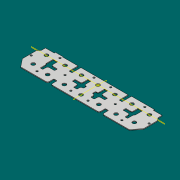
# Autodesk Inventor part: pcb_middle
Saved by Autodesk Inventor 2018 (Build 220112000, 112)
## iProperties
Created: 2021-10-17
Part Number: pcb_middle
Material: アルミニウム 6061
Document SubType Name: Modeling
Designer: gisen
Density: 2.7 g/cm^3
Appearance: アルミニウム - フラット
Author: gisen
Autodesk Inventor part; units mm, degrees
ref_plane "XY Plane" through (0, 0, 0) normal (0, 0, 1) x (1, 0, 0)
sketch "スケッチ1" plane through (0, 0, 0) normal (0, 0, 1) x (1, 0, 0)
  arc A0 (-25.2, 7.4139) -> (-26.2, 6.4139) centre (-25.2, 6.4139) ccw construction
  arc A1 (-19, 3.9139) -> (-21, 3.9139) centre (-20, 3.9139) ccw construction
  arc A2 (-10.8, 6.4139) -> (-11.8, 7.4139) centre (-11.8, 6.4139) ccw construction
  arc A3 (-6.7, 7.4139) -> (-7.7, 6.4139) centre (-6.7, 6.4139) ccw construction
  arc A4 (7.7, 6.4139) -> (6.7, 7.4139) centre (6.7, 6.4139) ccw construction
  arc A5 (11.8, 7.4139) -> (10.8, 6.4139) centre (11.8, 6.4139) ccw construction
  arc A6 (26.2, 6.4139) -> (25.2, 7.4139) centre (25.2, 6.4139) ccw construction
  line L0 (-67.1, -22.0601) -> (-67.1, -6.6726)
  line L1 (-67.1, -6.6726) -> (-64.6, -3.5297)
  line L2 (-64.6, -3.5297) -> (-64.6, 0.9639)
  line L3 (-64.6, 2.3139) -> (-54.9, 2.3139) construction
  line L4 (-29.4, 2.3139) -> (-29.4, 1.8139) construction
  line L5 (-28.8, -8.1959) -> (-26.7, -8.1959)
  line L6 (-26.1, -7.5959) -> (-26.1, 1.8139)
  line L7 (-26.1, 2.3139) -> (26.1, 2.3139) construction
  line L8 (26.1, 2.3139) -> (26.1, 1.8139)
  line L9 (26.7, -8.1959) -> (28.8, -8.1959)
  line L10 (29.4, -7.5959) -> (29.4, 2.3139)
  line L11 (29.4, 2.3139) -> (54.8, 2.3139)
  line L12 (64.6, 2.3139) -> (64.6, 0.9639) construction
  line L13 (64.6, -3.5297) -> (67.1, -6.6726)
  line L14 (67.1, -6.6726) -> (67.1, -22.0601)
  line L15 (67.1, -22.0601) -> (60.0795, -30.8861)
  line L16 (60.0795, -30.8861) -> (32, -30.8861)
  line L17 (30.3, -29.1861) -> (30.3, -24.5959)
  line L18 (29.7, -23.9959) -> (27.3, -23.9959)
  line L19 (26.7, -24.5959) -> (26.7, -29.1861)
  line L20 (25, -30.8861) -> (-25, -30.8861)
  line L21 (-26.7, -29.1861) -> (-26.7, -24.5959)
  line L22 (-27.3, -23.9959) -> (-29.7, -23.9959)
  line L23 (-30.3, -24.5959) -> (-30.3, -29.1861)
  line L24 (-32, -30.8861) -> (-60.0795, -30.8861)
  line L25 (-60.0795, -30.8861) -> (-67.1, -22.0601)
  line L26 (-64.5913, -25.214) -> (-66.9913, -22.1968) construction
  line L27 (64.5913, -25.214) -> (66.9913, -22.1968) construction
  line L28 (-66.0851, -5.2361) -> (-64.8087, -3.6314) construction
  line L29 (-67.1, -21.8855) -> (-67.1, -5.0802) construction
  line L30 (67.1, -5.0802) -> (67.1, -21.8855) construction
  line L31 (64.8087, -3.6314) -> (66.0851, -5.2361) construction
  line L32 (-45.0166, 2.4139) -> (-54.9, 2.4139) construction
  line L33 (54.8, 2.4139) -> (45.0166, 2.4139) construction
  arc A7 (-26.2, 0.8639) -> (-29.3, 0.8639) centre (-27.75, 0.8639) ccw construction
  line L34 (-45.0166, 2.4139) -> (-27.75, 2.4139) construction
  line L35 (-27.75, 2.4139) -> (-27.75, 0.8639) construction
  line L36 (-64.7, -3.3202) -> (-64.7, 0.0639) construction
  line L37 (64.7, 0.0639) -> (64.7, -3.3202) construction
  arc A8 (-32, -30.8861) -> (-30.3, -29.1861) centre (-32, -29.1861) ccw
  arc A9 (-26.7, -29.1861) -> (-25, -30.8861) centre (-25, -29.1861) ccw
  arc A10 (25, -30.8861) -> (26.7, -29.1861) centre (25, -29.1861) ccw
  arc A11 (30.3, -29.1861) -> (32, -30.8861) centre (32, -29.1861) ccw
  arc A12 (-32, -30.9861) -> (-30.2, -29.1861) centre (-32, -29.1861) ccw construction
  arc A13 (25, -31.2861) -> (26.8, -29.4861) centre (25, -29.4861) ccw construction
  arc A14 (30.2, -29.1861) -> (32, -30.9861) centre (32, -29.1861) ccw construction
  arc A15 (-26.8, -29.4861) -> (-25, -31.2861) centre (-25, -29.4861) ccw construction
  arc A16 (-29.7, -24.0959) -> (-30.2, -24.5959) centre (-29.7, -24.5959) ccw construction
  arc A17 (-26.8, -24.5959) -> (-27.3, -24.0959) centre (-27.3, -24.5959) ccw construction
  arc A18 (27.3, -24.0959) -> (26.8, -24.5959) centre (27.3, -24.5959) ccw construction
  arc A19 (30.2, -24.5959) -> (29.7, -24.0959) centre (29.7, -24.5959) ccw construction
  line L38 (-26.7, -8.0959) -> (-28.8, -8.0959) construction
  arc A20 (-29.4, -7.5959) -> (-28.8, -8.1959) centre (-28.8, -7.5959) ccw
  arc A21 (-26.7, -8.1959) -> (-26.1, -7.5959) centre (-26.7, -7.5959) ccw
  arc A22 (-29.3, -7.5959) -> (-28.8, -8.0959) centre (-28.8, -7.5959) ccw construction
  arc A23 (-26.7, -8.0959) -> (-26.2, -7.5959) centre (-26.7, -7.5959) ccw construction
  arc A24 (-29.7, -23.9959) -> (-30.3, -24.5959) centre (-29.7, -24.5959) ccw
  arc A25 (-26.7, -24.5959) -> (-27.3, -23.9959) centre (-27.3, -24.5959) ccw
  arc A26 (27.3, -23.9959) -> (26.7, -24.5959) centre (27.3, -24.5959) ccw
  arc A27 (30.3, -24.5959) -> (29.7, -23.9959) centre (29.7, -24.5959) ccw
  arc A28 (29.3, 0.8639) -> (26.2, 0.8639) centre (27.75, 0.8639) ccw construction
  arc A29 (26.2, -7.5959) -> (26.7, -8.0959) centre (26.7, -7.5959) ccw construction
  arc A30 (28.8, -8.0959) -> (29.3, -7.5959) centre (28.8, -7.5959) ccw construction
  arc A31 (26.1, -7.5959) -> (26.7, -8.1959) centre (26.7, -7.5959) ccw
  arc A32 (28.8, -8.1959) -> (29.4, -7.5959) centre (28.8, -7.5959) ccw
  line L39 (-26.1, 1.8139) -> (26.1, 1.8139)
  line L40 (-26.1, 1.8139) -> (-26.1, 2.3139) construction
  line L41 (26.1, 1.8139) -> (26.1, -7.5959)
  circle A33 centre (-47, -0.5861) radius 0.8 construction
  circle A34 centre (-65.2959, -14.0786) radius 0.8 construction
  circle A35 centre (-46.95, -25.9861) radius 0.8 construction
  circle A36 centre (-27.8915, -14.0959) radius 0.8 construction
  circle A37 centre (-9.25, -0.5861) radius 0.8 construction
  circle A38 centre (9.25, -0.5861) radius 0.8 construction
  circle A39 centre (27.8915, -14.0959) radius 0.8 construction
  circle A40 centre (9.55, -25.9861) radius 0.8 construction
  circle A41 centre (-9.55, -25.9861) radius 0.8 construction
  circle A42 centre (46.95, -25.9861) radius 0.8 construction
  circle A43 centre (47, -0.5861) radius 0.8 construction
  circle A44 centre (65.2959, -14.0786) radius 0.8 construction
  line L42 (-48.8, -5.4861) -> (-45.2, -5.4861)
  line L43 (-44.6, -6.0861) -> (-44.6, -10.7861)
  line L44 (-42.9, -12.4861) -> (-38.3915, -12.4861)
  line L45 (-37.7915, -13.0861) -> (-37.7915, -15.0861)
  line L46 (-38.3915, -15.6861) -> (-43.8, -15.6861)
  line L47 (-45.5, -17.3861) -> (-45.5, -20.4861)
  line L48 (-46.1, -21.0861) -> (-47.8, -21.0861)
  line L49 (-48.4, -20.4861) -> (-48.4, -15.2861)
  arc A45 (-48.4, -15.2861) -> (-49.1391, -13.8837) centre (-50.1, -15.2861) ccw
  arc A46 (-48.3, -15.2861) -> (-48.5711, -14.3361) centre (-50.1, -15.2861) ccw construction
  arc A47 (-49.4, -13.3887) -> (-49.1391, -13.8837) centre (-48.8, -13.3887) ccw
  line L50 (-49.4, -6.0861) -> (-49.4, -13.3887)
  arc A48 (-49.3, -13.3887) -> (-49.0826, -13.8012) centre (-48.8, -13.3887) ccw construction
  arc A49 (-48.8, -5.5861) -> (-49.3, -6.0861) centre (-48.8, -6.0861) ccw construction
  arc A50 (-44.7, -6.0861) -> (-45.2, -5.5861) centre (-45.2, -6.0861) ccw construction
  arc A51 (-44.7, -10.7861) -> (-44.5015, -11.6078) centre (-42.9, -10.7861) ccw construction
  arc A52 (-37.8915, -13.0861) -> (-38.3915, -12.5861) centre (-38.3915, -13.0861) ccw construction
  arc A53 (-38.3915, -15.5861) -> (-37.8915, -15.0861) centre (-38.3915, -15.0861) ccw construction
  arc A54 (-43.8, -15.5861) -> (-45.6, -17.3861) centre (-43.8, -17.3861) ccw construction
  arc A55 (-46.1, -20.9861) -> (-45.6, -20.4861) centre (-46.1, -20.4861) ccw construction
  arc A56 (-48.3, -20.4861) -> (-47.8, -20.9861) centre (-47.8, -20.4861) ccw construction
  arc A57 (-48.8, -5.4861) -> (-49.4, -6.0861) centre (-48.8, -6.0861) ccw
  arc A58 (-44.6, -6.0861) -> (-45.2, -5.4861) centre (-45.2, -6.0861) ccw
  arc A59 (-48.4, -20.4861) -> (-47.8, -21.0861) centre (-47.8, -20.4861) ccw
  arc A60 (-46.1, -21.0861) -> (-45.5, -20.4861) centre (-46.1, -20.4861) ccw
  arc A61 (-38.3915, -15.6861) -> (-37.7915, -15.0861) centre (-38.3915, -15.0861) ccw
  arc A62 (-37.7915, -13.0861) -> (-38.3915, -12.4861) centre (-38.3915, -13.0861) ccw
  arc A63 (-44.6, -10.7861) -> (-42.9, -12.4861) centre (-42.9, -10.7861) ccw
  arc A64 (-43.8, -15.6861) -> (-45.5, -17.3861) centre (-43.8, -17.3861) ccw
  arc A65 (-17.3915, -12.8861) -> (-17.8915, -13.3861) centre (-17.3915, -13.3861) ccw construction
  arc A66 (-17.8915, -15.3861) -> (-17.3915, -15.8861) centre (-17.3915, -15.3861) ccw construction
  arc A67 (-12.6, -12.8861) -> (-10.8984, -11.673) centre (-12.6, -11.0861) ccw construction
  arc A68 (-11.4, -17.6861) -> (-13.2, -15.8861) centre (-13.2, -17.6861) ccw construction
  arc A69 (-5.9, -16.4861) -> (-7.7, -18.2861) centre (-5.9, -18.2861) ccw construction
  arc A70 (-7.6652, -11.7382) -> (-5.9, -13.1861) centre (-5.9, -11.3861) ccw construction
  arc A71 (-10.3, -5.5861) -> (-10.8, -6.0861) centre (-10.3, -6.0861) ccw construction
  arc A72 (-7.7, -6.0861) -> (-8.2, -5.5861) centre (-8.2, -6.0861) ccw construction
  arc A73 (-5.5, -16.4861) -> (-5, -15.9861) centre (-5.5, -15.9861) ccw construction
  arc A74 (-5, -13.6861) -> (-5.5, -13.1861) centre (-5.5, -13.6861) ccw construction
  arc A75 (-8.2, -20.9861) -> (-7.7, -20.4861) centre (-8.2, -20.4861) ccw construction
  arc A76 (-11.4, -20.4861) -> (-10.9, -20.9861) centre (-10.9, -20.4861) ccw construction
  line L51 (-10.9, -11.0861) -> (-10.9, -6.0861)
  line L52 (-10.3, -5.4861) -> (-8.2, -5.4861)
  line L53 (-7.6, -6.0861) -> (-7.6, -11.3861)
  line L54 (-5.9, -13.0861) -> (-5.5, -13.0861)
  line L55 (-4.9, -13.6861) -> (-4.9, -15.9861)
  line L56 (-5.5, -16.5861) -> (-5.9, -16.5861)
  line L57 (-7.6, -18.2861) -> (-7.6, -20.4861)
  line L58 (-8.2, -21.0861) -> (-10.9, -21.0861)
  line L59 (-11.5, -20.4861) -> (-11.5, -17.6861)
  line L60 (-13.2, -15.9861) -> (-17.3915, -15.9861)
  line L61 (-17.9915, -15.3861) -> (-17.9915, -13.3861)
  line L62 (-17.3915, -12.7861) -> (-12.6, -12.7861)
  arc A77 (-11.5, -20.4861) -> (-10.9, -21.0861) centre (-10.9, -20.4861) ccw
  arc A78 (-8.2, -21.0861) -> (-7.6, -20.4861) centre (-8.2, -20.4861) ccw
  arc A79 (-5.5, -16.5861) -> (-4.9, -15.9861) centre (-5.5, -15.9861) ccw
  arc A80 (-4.9, -13.6861) -> (-5.5, -13.0861) centre (-5.5, -13.6861) ccw
  arc A81 (-7.6, -6.0861) -> (-8.2, -5.4861) centre (-8.2, -6.0861) ccw
  arc A82 (-10.3, -5.4861) -> (-10.9, -6.0861) centre (-10.3, -6.0861) ccw
  arc A83 (-17.3915, -12.7861) -> (-17.9915, -13.3861) centre (-17.3915, -13.3861) ccw
  arc A84 (-17.9915, -15.3861) -> (-17.3915, -15.9861) centre (-17.3915, -15.3861) ccw
  arc A85 (-12.6, -12.7861) -> (-10.9, -11.0861) centre (-12.6, -11.0861) ccw
  arc A86 (-7.6, -11.3861) -> (-5.9, -13.0861) centre (-5.9, -11.3861) ccw
  arc A87 (-5.9, -16.5861) -> (-7.6, -18.2861) centre (-5.9, -18.2861) ccw
  arc A88 (-11.5, -17.6861) -> (-13.2, -15.9861) centre (-13.2, -17.6861) ccw
  line L63 (0, 1.8139) -> (0, -30.8861) construction
  line L64 (48.8, -5.4861) -> (45.2, -5.4861)
  line L65 (44.6, -6.0861) -> (44.6, -10.7861)
  line L66 (42.9, -12.4861) -> (38.3915, -12.4861)
  line L67 (37.7915, -13.0861) -> (37.7915, -15.0861)
  line L68 (38.3915, -15.6861) -> (43.8, -15.6861)
  line L69 (45.5, -17.3861) -> (45.5, -20.4861)
  line L70 (46.1, -21.0861) -> (47.8, -21.0861)
  line L71 (48.4, -20.4861) -> (48.4, -15.2861)
  arc A89 (49.1391, -13.8837) -> (48.4, -15.2861) centre (50.1, -15.2861) ccw
  arc A90 (49.1391, -13.8837) -> (49.4, -13.3887) centre (48.8, -13.3887) ccw
  line L72 (49.4, -6.0861) -> (49.4, -13.3887)
  arc A91 (49.4, -6.0861) -> (48.8, -5.4861) centre (48.8, -6.0861) ccw
  arc A92 (45.2, -5.4861) -> (44.6, -6.0861) centre (45.2, -6.0861) ccw
  arc A93 (47.8, -21.0861) -> (48.4, -20.4861) centre (47.8, -20.4861) ccw
  arc A94 (45.5, -20.4861) -> (46.1, -21.0861) centre (46.1, -20.4861) ccw
  arc A95 (37.7915, -15.0861) -> (38.3915, -15.6861) centre (38.3915, -15.0861) ccw
  arc A96 (38.3915, -12.4861) -> (37.7915, -13.0861) centre (38.3915, -13.0861) ccw
  arc A97 (42.9, -12.4861) -> (44.6, -10.7861) centre (42.9, -10.7861) ccw
  arc A98 (45.5, -17.3861) -> (43.8, -15.6861) centre (43.8, -17.3861) ccw
  line L73 (10.9, -11.0861) -> (10.9, -6.0861)
  line L74 (10.3, -5.4861) -> (8.2, -5.4861)
  line L75 (7.6, -6.0861) -> (7.6, -11.3861)
  line L76 (5.9, -13.0861) -> (5.5, -13.0861)
  line L77 (4.9, -13.6861) -> (4.9, -15.9861)
  line L78 (7.6, -18.2861) -> (7.6, -20.4861)
  line L79 (8.2, -21.0861) -> (10.9, -21.0861)
  line L80 (11.5, -20.4861) -> (11.5, -17.6861)
  line L81 (13.2, -15.9861) -> (17.3915, -15.9861)
  line L82 (17.9915, -15.3861) -> (17.9915, -13.3861)
  line L83 (17.3915, -12.7861) -> (12.6, -12.7861)
  arc A99 (10.9, -21.0861) -> (11.5, -20.4861) centre (10.9, -20.4861) ccw
  arc A100 (7.6, -20.4861) -> (8.2, -21.0861) centre (8.2, -20.4861) ccw
  arc A101 (4.9, -15.9861) -> (5.5, -16.5861) centre (5.5, -15.9861) ccw
  arc A102 (5.5, -13.0861) -> (4.9, -13.6861) centre (5.5, -13.6861) ccw
  arc A103 (8.2, -5.4861) -> (7.6, -6.0861) centre (8.2, -6.0861) ccw
  arc A104 (10.9, -6.0861) -> (10.3, -5.4861) centre (10.3, -6.0861) ccw
  arc A105 (17.9915, -13.3861) -> (17.3915, -12.7861) centre (17.3915, -13.3861) ccw
  arc A106 (17.3915, -15.9861) -> (17.9915, -15.3861) centre (17.3915, -15.3861) ccw
  arc A107 (10.9, -11.0861) -> (12.6, -12.7861) centre (12.6, -11.0861) ccw
  arc A108 (5.9, -13.0861) -> (7.6, -11.3861) centre (5.9, -11.3861) ccw
  arc A109 (7.6, -18.2861) -> (5.9, -16.5861) centre (5.9, -18.2861) ccw
  arc A110 (13.2, -15.9861) -> (11.5, -17.6861) centre (13.2, -17.6861) ccw
  circle A111 centre (-65.2959, -14.0786) radius 1.05
  circle A112 centre (-47, -0.5861) radius 1.05
  circle A113 centre (-46.95, -25.9861) radius 1.05
  circle A114 centre (-27.8915, -14.0959) radius 1.05
  circle A115 centre (-9.25, -0.5861) radius 1.05
  circle A116 centre (-9.55, -25.9861) radius 1.05
  circle A117 centre (9.55, -25.9861) radius 1.05
  circle A118 centre (9.25, -0.5861) radius 1.05
  circle A119 centre (27.8915, -14.0959) radius 1.05
  circle A120 centre (46.95, -25.9861) radius 1.05
  circle A121 centre (47, -0.5861) radius 1.05
  circle A122 centre (65.2959, -14.0786) radius 1.05
  line L84 (5.5, -16.5861) -> (5.9, -16.5861)
  line L85 (-64.6, 0.9639) -> (-54.9, 0.9639)
  line L86 (-54.9, 0.9639) -> (-54.9, 2.3139)
  line L87 (-55, 14.0639) -> (-55, 2.7139) construction
  line L88 (-65.7, 1.0639) -> (-66.1, 1.0639) construction
  line L89 (-54.9, 2.3139) -> (-46.4, 2.3139)
  line L90 (-64.6, 0.9639) -> (-64.6, 2.3139) construction
  line L91 (54.9, 2.7139) -> (54.9, 11.2639) construction
  line L92 (66.1, 1.0639) -> (65.7, 1.0639) construction
  line L93 (54.8, 2.3139) -> (54.8, 0.9639)
  line L94 (54.8, 0.9639) -> (64.6, 0.9639)
  line L95 (54.8, 2.3139) -> (64.6, 2.3139) construction
  line L96 (64.6, 0.9639) -> (64.6, -3.5297)
  line L97 (-46.4, 2.3139) -> (-46.4, 1.8139)
  line L98 (-46.4, 1.8139) -> (-29.4, 1.8139)
  line L99 (-46.3, 14.0639) -> (-46.3, 3.1139) construction
  line L100 (-29.4, 1.8139) -> (-29.4, -7.5959)
  line L101 (-46.4, 2.3139) -> (-29.4, 2.3139) construction
  point P0 (0, 0)
  point P1 (26.7, -30.8861)
  point P2 (-26.7, -30.8861)
  point P3 (-30.3, -30.8861)
  dimension "d1" = 0.1
  dimension "d3" = 0.1
  dimension "d4" = 0.1
  dimension "d6" = 0.1
  dimension "d7" = 0.1
  dimension "d8" = 0.1
  dimension "d9" = 0.1
  dimension "d10" = 0.1
  dimension "d11" = 0.1
  dimension "d12" = 0.1
  dimension "d13" = 0.1
  dimension "d18" = 0.1
  dimension "d19" = 0.1
  dimension "d21" = 0.5
  dimension "d22" = 0.1
  dimension "d25" = 0.1
  dimension "d28" = 2.1
  dimension "d31" = 0.1
  dimension "d32" = 0.1
  dimension "d33" = 0.5
  dimension "d34" = 0.1
  dimension "d35" = 0.1
  dimension "d36" = 0.1
  constraints: 172 end point, 112 point on circle, 70 tangent, 68 centre point, 65 symmetric about line, 59 perpendicular, 34 equal radius, 33 coincident, 15 point on line, 9 vertical, 5 parallel, 4 horizontal, 2 collinear, 2 midpoint, 22 other
  measures "d1" distance from line of A16.end L23
  measures "d3" distance from line of L21 A17.start
  measures "d4" distance from line of L19 A18.end
  measures "d6" distance from line of A19.start L17
  measures "d7" distance from line of L28.start L1
  measures "d8" distance from line of L1.end L36
  measures "d9" distance from line of L3 L32.start
  measures "d10" distance from line of L37.start L12
  measures "d11" distance between parallel lines of L31 L13
  measures "d12" distance from line of A7.end L4
  measures "d13" distance from line of A7.start L6
  measures "d18" distance from line of A29.start L8
  measures "d19" distance from line of A30.end L10
  measures "d21" distance from line of L7 L6.end
  measures "d22" distance from line of L50 A49.end
  measures "d25" distance from line of L59 A76.start
  measures "d28" diameter of A111
  measures "d31" distance between parallel lines of L88 L85
  measures "d32" distance between parallel lines of L92 L94
  measures "d33" distance between parallel lines of L89 L98
  measures "d34" distance between parallel lines of L86 L87
  measures "d35" distance between parallel lines of L97 L99
  measures "d36" distance between parallel lines of L91 L93
extrude "押し出し1" add sketch "スケッチ1" along normal blind 0.8
sketch "スケッチ2" plane through (0, 0, 0.8) normal (0, 0, 1) x (1, 0, 0)
  arc A0 (-49.3, 0.4139) -> (-51.1, 2.2139) centre (-51.1, 0.4139) ccw construction
  arc A1 (-64.7, -11.3861) -> (-63.1942, -13.1618) centre (-62.9, -11.3861) ccw construction
  arc A2 (-63.0124, -13.8709) -> (-63.7, -15.2861) centre (-61.9, -15.2861) ccw construction
  arc A3 (-50.1, -28.8861) -> (-48.3, -27.0861) centre (-50.1, -27.0861) ccw construction
  arc A4 (-43.8, -15.5861) -> (-45.6, -17.3861) centre (-43.8, -17.3861) ccw construction
  arc A5 (-32, -30.9861) -> (-30.2, -29.1861) centre (-32, -29.1861) ccw construction
  arc A6 (-25, -15.8861) -> (-26.8, -17.6861) centre (-25, -17.6861) ccw construction
  arc A7 (-13.2, -31.2861) -> (-11.4, -29.4861) centre (-13.2, -29.4861) ccw construction
  arc A8 (-5.9, -16.4861) -> (-7.7, -18.2861) centre (-5.9, -18.2861) ccw construction
  arc A9 (6.6435, -31.7253) -> (7.7, -30.0861) centre (5.9, -30.0861) ccw construction
  arc A10 (-29.3, 1.0139) -> (-29.3522, 1.4444) centre (-31.1, 1.0139) ccw construction
  arc A11 (-44.5015, -11.6078) -> (-42.9, -12.5861) centre (-42.9, -10.7861) ccw construction
  arc A12 (-26.1016, -11.673) -> (-24.4, -12.8861) centre (-24.4, -11.0861) ccw construction
  arc A13 (-10.9274, 1.3792) -> (-12.6, 2.5139) centre (-12.6, 0.7139) ccw construction
  arc A14 (-7.4588, 1.3139) -> (-7.7, 0.4139) centre (-5.9, 0.4139) ccw construction
  arc A15 (5.9, -13.1861) -> (7.6652, -11.7382) centre (5.9, -11.3861) ccw construction
  arc A16 (10.9274, 1.3792) -> (10.8, 0.7139) centre (12.6, 0.7139) ccw construction
  arc A17 (26.1016, -11.673) -> (26.2, -11.0861) centre (24.4, -11.0861) ccw construction
  arc A18 (31.1, 2.8139) -> (29.3522, 1.4444) centre (31.1, 1.0139) ccw construction
  arc A19 (44.5015, -11.6078) -> (44.7, -10.7861) centre (42.9, -10.7861) ccw construction
  arc A20 (51.1, 2.2139) -> (49.3, 0.4139) centre (51.1, 0.4139) ccw construction
  arc A21 (63.1942, -13.1618) -> (64.7, -11.3861) centre (62.9, -11.3861) ccw construction
  arc A22 (48.3, -27.0861) -> (49.825, -28.8649) centre (50.1, -27.0861) ccw construction
  arc A23 (63.7, -15.2861) -> (63.0124, -13.8709) centre (61.9, -15.2861) ccw construction
  arc A24 (45.6, -17.3861) -> (43.8, -15.5861) centre (43.8, -17.3861) ccw construction
  arc A25 (15.8, -58.8861) -> (15.2, -58.2861) centre (15.2, -58.8861) ccw construction
  line L0 (15.8, -58.8861) -> (15.8, -62.2861) construction
  arc A26 (15.2, -62.8861) -> (15.8, -62.2861) centre (15.2, -62.2861) ccw construction
  line L1 (15.2, -62.8861) -> (8.2, -62.8861) construction
  arc A27 (7.6, -62.2861) -> (8.2, -62.8861) centre (8.2, -62.2861) ccw construction
  line L2 (7.6, -62.2861) -> (7.6, -58.8861) construction
  arc A28 (8.2, -58.2861) -> (7.6, -58.8861) centre (8.2, -58.8861) ccw construction
  line L3 (8.2, -58.2861) -> (15.2, -58.2861) construction
  arc A29 (-7.6, -58.8861) -> (-8.2, -58.2861) centre (-8.2, -58.8861) ccw construction
  line L4 (-7.6, -58.8861) -> (-7.6, -62.2861) construction
  arc A30 (-8.2, -62.8861) -> (-7.6, -62.2861) centre (-8.2, -62.2861) ccw construction
  line L5 (-8.2, -62.8861) -> (-15.2, -62.8861) construction
  arc A31 (-15.8, -62.2861) -> (-15.2, -62.8861) centre (-15.2, -62.2861) ccw construction
  line L6 (-15.8, -62.2861) -> (-15.8, -58.8861) construction
  arc A32 (-15.2, -58.2861) -> (-15.8, -58.8861) centre (-15.2, -58.8861) ccw construction
  line L7 (-15.2, -58.2861) -> (-8.2, -58.2861) construction
  arc A33 (-3.85, -54.4861) -> (-3.25, -55.0861) centre (-3.25, -54.4861) ccw construction
  line L8 (-3.85, -54.4861) -> (-3.85, -53.2461) construction
  arc A34 (-3.25, -52.6461) -> (-3.85, -53.2461) centre (-3.25, -53.2461) ccw construction
  line L9 (-3.25, -52.6461) -> (3.25, -52.6461) construction
  arc A35 (3.85, -53.2461) -> (3.25, -52.6461) centre (3.25, -53.2461) ccw construction
  line L10 (3.85, -53.2461) -> (3.85, -54.4861) construction
  arc A36 (3.25, -55.0861) -> (3.85, -54.4861) centre (3.25, -54.4861) ccw construction
  line L11 (3.25, -55.0861) -> (-3.25, -55.0861) construction
  circle A37 centre (30.05, -39.9861) radius 1.05 construction
  circle A38 centre (38.492, -53.6861) radius 1.05 construction
  circle A39 centre (11.7, -65.7861) radius 1.05 construction
  circle A40 centre (9.75, -53.1361) radius 1.05 construction
  circle A41 centre (-9.75, -53.1361) radius 1.05 construction
  circle A42 centre (-11.7, -65.7861) radius 1.05 construction
  circle A43 centre (-38.492, -53.6861) radius 1.05 construction
  circle A44 centre (-30.05, -39.9861) radius 1.05 construction
  line L12 (-27.3621, -37.0861) -> (-32.4, -37.0861) construction
  arc A45 (-33, -36.4861) -> (-32.4, -37.0861) centre (-32.4, -36.4861) ccw construction
  line L13 (-33, -36.4861) -> (-33, -31.3861) construction
  arc A46 (-33, -31.3861) -> (-33.9, -30.4861) centre (-33.9, -31.3861) ccw construction
  line L14 (-33.9, -30.4861) -> (-44.6, -30.4861) construction
  arc A47 (-44.6, -30.4861) -> (-45.5, -31.3861) centre (-44.6, -31.3861) ccw construction
  line L15 (-45.5, -31.3861) -> (-45.5, -34.7861) construction
  arc A48 (-46.1, -35.3861) -> (-45.5, -34.7861) centre (-46.1, -34.7861) ccw construction
  line L16 (-46.1, -35.3861) -> (-46.5, -35.3861) construction
  arc A49 (-46.5, -35.3861) -> (-48.2, -37.0861) centre (-46.5, -37.0861) ccw construction
  line L17 (-48.2, -37.0861) -> (-48.2, -48.8861) construction
  arc A50 (-48.2, -48.8861) -> (-46.5, -50.5861) centre (-46.5, -48.8861) ccw construction
  line L18 (-46.5, -50.5861) -> (-46.1031, -50.5861) construction
  arc A51 (-45.6678, -50.773) -> (-46.1031, -50.5861) centre (-46.1031, -51.1861) ccw construction
  line L19 (-45.6678, -50.773) -> (-31, -66.2297) construction
  line L20 (-31, -66.2297) -> (-31, -68.4088) construction
  line L21 (-31, -68.4088) -> (-29.788, -69.6861) construction
  line L22 (-29.788, -69.6861) -> (-7.1961, -69.6861) construction
  arc A52 (-7.1961, -69.6861) -> (-5.9, -70.2861) centre (-5.9, -68.5861) ccw construction
  line L23 (-5.9, -70.2861) -> (5.9, -70.2861) construction
  arc A53 (5.9, -70.2861) -> (7.1961, -69.6861) centre (5.9, -68.5861) ccw construction
  line L24 (7.1961, -69.6861) -> (29.788, -69.6861) construction
  line L25 (29.788, -69.6861) -> (31, -68.4088) construction
  line L26 (31, -68.4088) -> (31, -66.2297) construction
  line L27 (31, -66.2297) -> (45.6678, -50.773) construction
  arc A54 (46.1031, -50.5861) -> (45.6678, -50.773) centre (46.1031, -51.1861) ccw construction
  line L28 (46.1031, -50.5861) -> (46.5, -50.5861) construction
  arc A55 (46.5, -50.5861) -> (48.2, -48.8861) centre (46.5, -48.8861) ccw construction
  line L29 (48.2, -48.8861) -> (48.2, -37.0861) construction
  arc A56 (48.2, -37.0861) -> (46.5, -35.3861) centre (46.5, -37.0861) ccw construction
  line L30 (46.5, -35.3861) -> (46.1, -35.3861) construction
  arc A57 (45.5, -34.7861) -> (46.1, -35.3861) centre (46.1, -34.7861) ccw construction
  line L31 (45.5, -34.7861) -> (45.5, -31.3861) construction
  arc A58 (45.5, -31.3861) -> (44.6, -30.4861) centre (44.6, -31.3861) ccw construction
  line L32 (44.6, -30.4861) -> (33.9, -30.4861) construction
  arc A59 (33.9, -30.4861) -> (33, -31.3861) centre (33.9, -31.3861) ccw construction
  line L33 (33, -31.3861) -> (33, -36.4861) construction
  arc A60 (32.4, -37.0861) -> (33, -36.4861) centre (32.4, -36.4861) ccw construction
  line L34 (32.4, -37.0861) -> (27.3621, -37.0861) construction
  arc A61 (26.8503, -36.7991) -> (27.3621, -37.0861) centre (27.3621, -36.4861) ccw construction
  arc A62 (26.8503, -36.7991) -> (25.4, -35.9861) centre (25.4, -37.6861) ccw construction
  line L35 (25.4, -35.9861) -> (13.6, -35.9861) construction
  arc A63 (13.6, -35.9861) -> (11.9, -37.6861) centre (13.6, -37.6861) ccw construction
  line L36 (11.9, -37.6861) -> (11.9, -42.6361) construction
  arc A64 (11.3, -43.2361) -> (11.9, -42.6361) centre (11.3, -42.6361) ccw construction
  line L37 (11.3, -43.2361) -> (8.2, -43.2361) construction
  arc A65 (7.6, -42.6361) -> (8.2, -43.2361) centre (8.2, -42.6361) ccw construction
  line L38 (7.6, -42.6361) -> (7.6, -39.1461) construction
  arc A66 (7.6, -39.1461) -> (6.7804, -37.6918) centre (5.9, -39.1461) ccw construction
  arc A67 (6.25, -36.7507) -> (6.7804, -37.6918) centre (7.35, -36.7507) ccw construction
  line L39 (6.25, -36.7507) -> (6.25, -31.3861) construction
  arc A68 (6.25, -31.3861) -> (5.35, -30.4861) centre (5.35, -31.3861) ccw construction
  line L40 (5.35, -30.4861) -> (-5.35, -30.4861) construction
  arc A69 (-5.35, -30.4861) -> (-6.25, -31.3861) centre (-5.35, -31.3861) ccw construction
  line L41 (-6.25, -31.3861) -> (-6.25, -36.7507) construction
  arc A70 (-6.7804, -37.6918) -> (-6.25, -36.7507) centre (-7.35, -36.7507) ccw construction
  arc A71 (-6.7804, -37.6918) -> (-7.6, -39.1461) centre (-5.9, -39.1461) ccw construction
  line L42 (-7.6, -39.1461) -> (-7.6, -42.6361) construction
  arc A72 (-8.2, -43.2361) -> (-7.6, -42.6361) centre (-8.2, -42.6361) ccw construction
  line L43 (-8.2, -43.2361) -> (-11.3, -43.2361) construction
  arc A73 (-11.9, -42.6361) -> (-11.3, -43.2361) centre (-11.3, -42.6361) ccw construction
  line L44 (-11.9, -42.6361) -> (-11.9, -37.6861) construction
  arc A74 (-11.9, -37.6861) -> (-13.6, -35.9861) centre (-13.6, -37.6861) ccw construction
  line L45 (-13.6, -35.9861) -> (-25.4, -35.9861) construction
  arc A75 (-25.4, -35.9861) -> (-26.8503, -36.7991) centre (-25.4, -37.6861) ccw construction
  arc A76 (-27.3621, -37.0861) -> (-26.8503, -36.7991) centre (-27.3621, -36.4861) ccw construction
  arc A77 (30.2, -29.1861) -> (32, -30.9861) centre (32, -29.1861) ccw construction
  arc A78 (26.8, -17.6861) -> (25, -15.8861) centre (25, -17.6861) ccw construction
  arc A79 (11.4, -29.4861) -> (13.2, -31.2861) centre (13.2, -29.4861) ccw construction
  line L46 (61.9, -15.2861) -> (50.1, -27.0861) construction
  line L47 (43.8, -17.3861) -> (32, -29.1861) construction
  line L48 (25, -17.6861) -> (13.2, -29.4861) construction
  line L49 (-5.9, -18.2861) -> (5.9, -30.0861) construction
  line L50 (-25, -17.6861) -> (-13.2, -29.4861) construction
  line L51 (-43.8, -17.3861) -> (-32, -29.1861) construction
  line L52 (-61.9, -15.2861) -> (-50.1, -27.0861) construction
  line L53 (-62.9, -11.3861) -> (-51.1, 0.4139) construction
  line L54 (-42.9, -10.7861) -> (-31.1, 1.0139) construction
  line L55 (-24.4, -11.0861) -> (-12.6, 0.7139) construction
  line L56 (-5.9, 0.4139) -> (5.9, -11.3861) construction
  line L57 (12.6, 0.7139) -> (24.4, -11.0861) construction
  line L58 (31.1, 1.0139) -> (42.9, -10.7861) construction
  line L59 (51.1, 0.4139) -> (62.9, -11.3861) construction
  circle A80 centre (-57, -5.4861) radius 2
  circle A81 centre (-37, -4.8861) radius 2
  circle A82 centre (-18.5, -5.1861) radius 2
  circle A83 centre (0, -5.4861) radius 2
  circle A84 centre (18.5, -5.1861) radius 2
  circle A85 centre (37, -4.8861) radius 2
  circle A86 centre (57, -5.4861) radius 2
  circle A87 centre (56, -21.1861) radius 2
  circle A88 centre (37.9, -23.2861) radius 2
  circle A89 centre (19.1, -23.5861) radius 2
  circle A90 centre (0, -24.1861) radius 2
  circle A91 centre (-19.1, -23.5861) radius 2
  circle A92 centre (-37.9, -23.2861) radius 2
  circle A93 centre (-56, -21.1861) radius 2
  circle A94 centre (0, -62.6861) radius 2 projected
  circle A95 centre (40.6, -42.9861) radius 2 projected
  circle A96 centre (0, -45.0461) radius 2 projected
  circle A97 centre (-40.6, -42.9861) radius 2 projected
  circle A98 centre (-19.5, -43.5861) radius 2 projected
  circle A99 centre (19.5, -43.5861) radius 2 projected
  circle A100 centre (23.4, -62.0861) radius 2 projected
  circle A101 centre (-23.4, -62.0861) radius 2 projected
  line L60 (27.7, -45.8861) -> (32.4, -45.8861) projected
  arc A102 (33, -46.4861) -> (32.4, -45.8861) centre (32.4, -46.4861) ccw projected
  line L61 (33, -46.4861) -> (33, -48.8861) projected
  arc A103 (33, -48.8861) -> (34.4806, -50.5718) centre (34.7, -48.8861) ccw projected
  arc A104 (34.8384, -51.5798) -> (34.4806, -50.5718) centre (34.4032, -51.1668) ccw projected
  line L62 (34.8384, -51.5798) -> (31.4883, -55.1102) projected
  arc A105 (30.5957, -55.0856) -> (31.4883, -55.1102) centre (31.0531, -54.6972) ccw projected
  arc A106 (30.5957, -55.0856) -> (29.3, -54.4861) centre (29.3, -56.1861) ccw projected
  line L63 (29.3, -54.4861) -> (22.2, -54.4861) projected
  arc A107 (21.6, -53.8861) -> (22.2, -54.4861) centre (22.2, -53.8861) ccw projected
  line L64 (21.6, -53.8861) -> (21.6, -51.7861) projected
  arc A108 (22.2, -51.1861) -> (21.6, -51.7861) centre (22.2, -51.7861) ccw projected
  line L65 (22.2, -51.1861) -> (25.4, -51.1861) projected
  arc A109 (25.4, -51.1861) -> (27.1, -49.4861) centre (25.4, -49.4861) ccw projected
  line L66 (27.1, -49.4861) -> (27.1, -46.4861) projected
  arc A110 (27.7, -45.8861) -> (27.1, -46.4861) centre (27.7, -46.4861) ccw projected
  line L67 (-27.1, -46.4861) -> (-27.1, -49.4861) projected
  arc A111 (-27.1, -49.4861) -> (-25.4, -51.1861) centre (-25.4, -49.4861) ccw projected
  line L68 (-25.4, -51.1861) -> (-22.2, -51.1861) projected
  arc A112 (-21.6, -51.7861) -> (-22.2, -51.1861) centre (-22.2, -51.7861) ccw projected
  line L69 (-21.6, -51.7861) -> (-21.6, -53.8861) projected
  arc A113 (-22.2, -54.4861) -> (-21.6, -53.8861) centre (-22.2, -53.8861) ccw projected
  line L70 (-22.2, -54.4861) -> (-29.3, -54.4861) projected
  arc A114 (-29.3, -54.4861) -> (-30.5957, -55.0856) centre (-29.3, -56.1861) ccw projected
  arc A115 (-31.4883, -55.1102) -> (-30.5957, -55.0856) centre (-31.0531, -54.6972) ccw projected
  line L71 (-31.4883, -55.1102) -> (-34.8384, -51.5798) projected
  arc A116 (-34.4806, -50.5718) -> (-34.8384, -51.5798) centre (-34.4032, -51.1668) ccw projected
  arc A117 (-34.4806, -50.5718) -> (-33, -48.8861) centre (-34.7, -48.8861) ccw projected
  line L72 (-33, -48.8861) -> (-33, -46.4861) projected
  arc A118 (-32.4, -45.8861) -> (-33, -46.4861) centre (-32.4, -46.4861) ccw projected
  line L73 (-32.4, -45.8861) -> (-27.7, -45.8861) projected
  arc A119 (-27.1, -46.4861) -> (-27.7, -45.8861) centre (-27.7, -46.4861) ccw projected
  point P0 (0, 0)
  dimension "d37" = 4
  constraints: 28 end point, 14 centre point, 14 midpoint, 13 equal radius
  measures "d37" diameter of A80
extrude "押し出し2" cut sketch "スケッチ2" against normal through all contours A80 | A81 | A82 | A83 | A84 | A85 | A86 | A87 | A88 | A89 | A90 | A91 | A92 | A93
ref_plane "作業平面2" through (0, -5.486, 0) normal (0, 1, 0) x (-1, 0, 0)
ref_plane "作業平面1" through (0, -0.086, 0) normal (0, 1, 0) x (-1, 0, 0)
equation "\"d3\" = d1"
equation "\"d4\" = d1"
equation "\"d6\" = d1"
equation "\"d7\" = d1"
equation "\"d8\" = d1"
equation "\"d9\" = d1"
equation "\"d10\" = d1"
equation "\"d11\" = d1"
equation "\"d12\" = d1"
equation "\"d13\" = d1"
equation "\"d18\" = d1"
equation "\"d19\" = d1"
equation "\"d22\" = d1"
equation "\"d25\" = d1"
equation "\"d31\" = d1"
equation "\"d32\" = d1"
equation "\"d34\" = d1"
equation "\"d35\" = d1"
equation "\"d36\" = d1"
